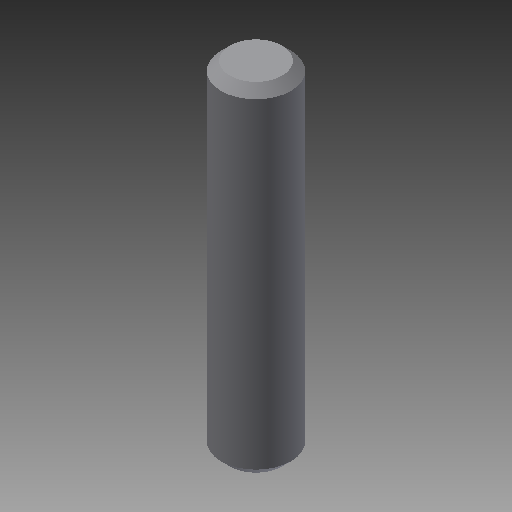
# Autodesk Inventor part: 4489_pin
Saved by Autodesk Inventor 2019 (Build 230136000, 136)
## iProperties
Category: PARTsolutions
Company: 8020
Created: 2019-03-04
Part Number: 4489_pin
Material: Generic
Catalog Web Link: www.cadenas.de
Description: 4488, 4489_pin-Combination Hinges
Vendor: 8020
Document SubType Name: Modeling
Designer: psadmin
Manufacturer: 8020
Mass: 2.11508 g
Surface Area: 11.0993 cm^2
Volume: 2.11508 cm^3
Density: 1 g/cm^3
Appearance: PSOLRGB-192-192-192
PSOL_IDENT_0: {$CADENAS_DATA\23d-libs\8020\inch\panels_and_doors\4488_pin.prj},166 {VTYP=3D},{NB=4489_pin},{LINA=4
PSOL_IDENT_1: 489_pin},{NN=4488, 4489_pin},{DATE=04.12.2018 10:30:19},{GEOMDATE=01.02.2012 11:10:00},{VERSION=},{L
PSOL_IDENT_2: INEID=10},{WBVAR=TS},{WBNUMERIC=}  {NB=4489_pin},{LINA=4489_pin},{KT=DUMMY},{PN=4489},{TS=Without Ha
PSOL_IDENT_3: ndle},{B=1.57480315}
NN: 4488, 4489_pin
NT: Combination Hinges
NB: 4489_pin
NBSYN: $PN._pin
LINA: 4489_pin
PN: 4489
TS: Without Handle
B: 1.57480315
SUPPLIER: 8020
ARTICLENO: 4489_pin
BOMINFO: 4489_pin
CREATOR: CADENAS GmbH
Title: 4489_pin
Author: Cadenas PARTsolutions
Comments: Combination Hinges
Autodesk Inventor part; units mm, degrees
sketch "Sketch_1" plane through (0, 0, 0) normal (0, 0, 1) x (1, 0, 0)
  line L0 (0, -20) -> (0, 20)
  line L1 (0, 20) -> (3.0861, 20)
  line L2 (3.0861, 20) -> (4.1275, 18.9586)
  line L3 (4.1275, 18.9586) -> (4.1275, -18.9586)
  line L4 (4.1275, -18.9586) -> (3.0861, -20)
  line L5 (3.0861, -20) -> (0, -20)
  line L6 (0, -20) -> (0, 20)
  constraints: 14 end point
revolve "Revolution1" add sketch "Sketch_1" angle 360 about axis through (0, -20, 0) along (0, -1, 0)
ref_plane "to_a_XY" through (0, 0, 0) normal (0, 1, 0) x (1, 0, 0)
ref_plane "to_a_YZ" through (0, 0, 0) normal (1, 0, 0) x (0, 0, -1)
ref_plane "to_a_ZX" through (0, 0, 0) normal (0, 0, -1) x (0, 1, 0)
body "Solid1"
